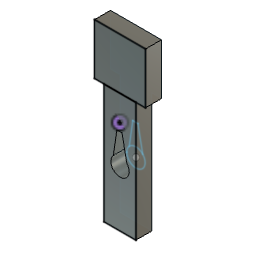
deciding the arm and placement of propellers with tyre rim (Autodesk Fusion 360 archive; units mm, degrees)
design "Untitled"
Autodesk Fusion 360 part; units mm, degrees
sketch "Sketch1" plane through (0, 0, 0) normal (0, 1, 0) x (1, 0, 0)
  line L0 (-16, -48) -> (16, -48)
  line L1 (16, -48) -> (16, -16)
  line L2 (16, -16) -> (-16, -16)
  line L3 (-16, -16) -> (-16, -48)
  line L4 (-10, -16) -> (10, -16)
  line L5 (10, -16) -> (10, 59)
  line L6 (10, 59) -> (-10, 59)
  line L7 (-10, 59) -> (-10, -16)
  dimension "d1" = 32
  dimension "d2" = 32
  dimension "d3" = 16
  dimension "d4" = 16
  dimension "d5" = 75
  dimension "d6" = 20
  dimension "d7" = 10
  constraint horizontal L0
  constraint vertical L1
  constraint horizontal L2
  constraint vertical L3
  constraint horizontal L4
  constraint vertical L5
  constraint horizontal L6
  constraint vertical L7
  constraint coincident L2 L4.start
  measures "d1" distance of L0.start L2.end
  measures "d2" distance of L0.start L0.end
  measures "d3" distance of origin L2
  measures "d4" distance of origin L3
  measures "d5" distance of L4.start L6.end
  measures "d6" distance of L5 L7
  measures "d7" distance of origin L5
extrude "Extrude1" add sketch "Sketch1" along normal blind 10
sketch "Sketch2" plane through (0, 10, 0) normal (0, 1, 0) x (-1, 0, 0)
  line L0 (10, -59) -> (10, 16)
  line L1 (10, 16) -> (16, 16)
  line L2 (16, 16) -> (16, 48)
  line L3 (16, 48) -> (-16, 48)
  line L4 (-16, 48) -> (-16, 16)
  line L5 (-16, 16) -> (-10, 16)
  line L6 (-10, 16) -> (-10, -59)
  line L7 (-10, -59) -> (10, -59)
  circle A0 centre (0, -24) radius 5.75
  line L8 (4.2156, -20.0896) -> (2, -5)
  line L9 (2, -5) -> (-1.2451, -5)
  line L10 (-1.2451, -5) -> (-4.2458, -20.1224)
  dimension "d10" = 11.5
  constraint coincident A0 L8.start
  constraint horizontal L9
  constraint coincident A0 L10.end
  measures "d10" diameter of A0
extrude "Extrude2" cut sketch "Sketch2" against normal blind 10 contours A0 | A0 L8 L9 L10
